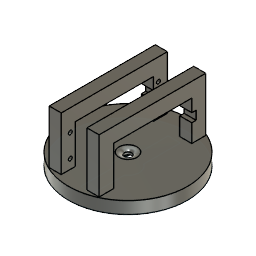
Circle (Autodesk Fusion 360 design; units mm, degrees)
Autodesk Fusion 360 part; units mm, degrees
sketch "Sketch1" plane through (0, 0, 0) normal (0, 0, 1) x (1, 0, 0)
  circle A0 centre (0, 0) radius 31.115
  dimension "d1" = 62.23
  constraint coincident A0.centre origin
  measures "d1" diameter of A0
extrude "Extrude1" add sketch "Sketch1" along normal blind 7.62 contours A0 picked at (8.859186, 0.873231) makes body 1
sketch "Sketch2" plane through (0, 0, 7.62) normal (0, 0, 1) x (-1, 0, 0)
  circle A0 centre (0, 0) radius 31.115
  circle A1 centre (0, 0) radius 1.905
  dimension "d4" = 3.81
  constraint coincident A0.centre A1.centre
  measures "d4" diameter of A1
extrude "Extrude2" cut sketch "Sketch2" against normal blind 27.94 contours A1 picked at (-0.336742, 0.293155) bodies 1
extrude "Extrude3" cut 1 faces at (21.255398, -1.640459, 7.62) along direction (0, 0, -1) blind 1.27 on bodies 1 bodies 1
sketch "Sketch3" plane through (0, 0, 6.35) normal (0, 0, 1) x (-1, 0, 0)
  circle A0 centre (0, 0) radius 1.905
  circle A1 centre (0, 0) radius 31.115
  line L0 (3.173876, -26.67) -> (-3.176124, -26.67)
  line L1 (3.173876, -26.67) -> (3.173876, 24.13)
  line L2 (-3.176124, -26.67) -> (-3.176124, 21.675024)
  line L3 (3.173876, 24.13) -> (-3.176124, 24.13)
  line L4 (-3.176124, 24.13) -> (-3.176124, 21.675024)
  dimension "d9" = 50.8
  constraint horizontal L0
  constraint perpendicular L0 L1
  constraint perpendicular L0 L2
  constraint perpendicular L2 L3
  constraint perpendicular L3 L4
extrude "Extrude4" cut sketch "Sketch3" against normal blind 5.08 contours L0 L1 L2 L3 L4 picked at (-0.048203, -18.413224) bodies 1
sketch "Sketch4" plane through (0, 0, 6.35) normal (0, 0, 1) x (-1, 0, 0)
  line L0 (-3.176124, 24.13) -> (3.173876, 24.13)
  line L1 (3.173876, 24.13) -> (3.173876, -26.67)
  line L2 (3.173876, -26.67) -> (-3.176124, -26.67)
  line L3 (-3.176124, -26.67) -> (-3.176124, 24.13)
  circle A0 centre (0, 0) radius 31.115
  circle A1 centre (0, 0) radius 5.08
  constraint coincident A0.centre A1.centre
extrude "Extrude5" cut sketch "Sketch4" against normal blind 5.08 contours L3 A1 | L1 A1 picked at (-4.180187, 0) picked at (3.3588, -1.150052) bodies 1
extrude "Extrude6" cut 1 faces at (-3.173876, -10.687649, 4.656667) along direction (-1, 0, 0) blind 2.54 on bodies 1 bodies 1
extrude "Extrude7" cut 1 faces at (-3.173876, 11.534316, 2.963333) along direction (-1, 0, 0) blind 2.54 on bodies 1 bodies 1
extrude "Extrude8" cut 1 faces at (3.176124, 19.101558, 4.656667) along direction (1, 0, 0) blind 2.54 on bodies 1 bodies 1
extrude "Extrude9" cut 1 faces at (3.176124, -17.408225, 4.656667) along direction (1, 0, 0) blind 2.54 on bodies 1 bodies 1
sketch "Sketch5" plane through (0, 0, 6.35) normal (0, 0, 1) x (-1, 0, 0)
  circle A0 centre (0, 0) radius 31.115
  line L0 (-3.176124, 3.964673) -> (-5.716124, 3.964673)
  line L1 (-5.716124, 3.964673) -> (-5.716124, 24.13)
  line L2 (-5.716124, 24.13) -> (5.713876, 24.13)
  line L3 (5.713876, 24.13) -> (5.713876, 3.966474)
  line L4 (5.713876, 3.966474) -> (3.173876, 3.966474)
  arc A1 (3.173876, -3.966474) -> (3.173876, 3.966474) centre (0, 0) ccw
  line L5 (3.173876, -3.966474) -> (5.713876, -3.966474)
  line L6 (5.713876, -3.966474) -> (5.713876, -26.67)
  line L7 (5.713876, -26.67) -> (-5.716124, -26.67)
  line L8 (-5.716124, -26.67) -> (-5.716124, -3.964673)
  line L9 (-5.716124, -3.964673) -> (-3.176124, -3.964673)
  arc A2 (-3.176124, 3.964673) -> (-3.176124, -3.964673) centre (0, 0) ccw
  circle A3 centre (0, 0) radius 7.62
  constraint coincident A0.centre A1.centre
extrude "Extrude10" cut sketch "Sketch5" against normal blind 5.08 contours L0 L1 L8 L9 A2 A3 | L3 L4 A1 L5 L6 A3 picked at (-5.736875, 3.121518) picked at (5.735631, -3.123168) bodies 1
extrude "Extrude11" add 1 faces at (1.906124, 26.67, 2.963333) along direction (0, -1, 0) blind 2.54 on bodies 1 bodies 1
extrude "Extrude12" add 1 faces at (-1.903876, -24.13, 2.963333) along direction (0, 1, 0) blind 2.54 on bodies 1 bodies 1
move_body "Move1" bodies 1 to x (-1, 0, 0) y (0, 1, 0) z (0, 0, -1) at (24.534657, 0, 12.7)
extrude "Extrude13" add 1 faces at (30.248533, -10.557621, 8.043333) along direction (-1, 0, 0) blind 0.127 on bodies 1 bodies 1
extrude "Extrude14" add 1 faces at (30.248533, 17.767144, 8.043333) along direction (-1, 0, 0) blind 0.127 on bodies 1 bodies 1
extrude "Extrude15" add 1 faces at (18.818533, 11.402588, 9.736666) along direction (1, 0, 0) blind 0.127 on bodies 1 bodies 1
extrude "Extrude16" add 1 faces at (18.818533, -16.072961, 9.736666) along direction (1, 0, 0) blind 0.127 on bodies 1 bodies 1
sketch "Sketch6" plane through (0, 0, 0) normal (1, 0, 0) x (0, 1, 0)
sketch "Sketch7" plane through (0, 0, 0) normal (1, 0, 0) x (0, 1, 0)
move_body "Move2" bodies 1 to x (1, 0, 0) y (0, 1, 0) z (0, 0, 1) at (-20.32, 0, -7.62)
sketch "Sketch9" plane through (0, 0, 0) normal (0, 1, 0) x (1, 0, 0)
sketch "Sketch10" plane through (0, 0, 0) normal (0, 1, 0) x (1, 0, 0)
sketch "Sketch11" plane through (0, 0, 0) normal (0, 1, 0) x (1, 0, 0)
sketch "Sketch12" plane through (0, 0, 0) normal (0, 1, 0) x (1, 0, 0)
  line L0 (0, -38.100001) -> (40.894, -38.100001)
  line L1 (40.894, -38.100001) -> (40.894, -17.526001)
  line L2 (40.894, -17.526001) -> (0, -17.526001)
  line L3 (0, -17.526001) -> (0, -38.100001)
  circle A0 centre (20.447, -27.813001) radius 27.94
  dimension "d39" = 40.894
  dimension "d40" = 20.574
  dimension "d41" = 55.88
  constraint horizontal L0
  constraint vertical L1
  constraint horizontal L2
  constraint vertical L3
  measures "d41" diameter of A0
move_body "Move3" bodies 1 to x (1, 0, 0) y (0, 1, 0) z (0, 0, 1) at (-55.88, 0, 0)
sketch "Sketch13" plane through (0, 0, 0) normal (1, 0, 0) x (0, 1, 0)
sketch "Sketch14" plane through (0, 0, 0) normal (1, 0, 0) x (0, 1, 0)
sketch "Sketch15" plane through (0, 0, 0) normal (1, 0, 0) x (0, 1, 0)
  line L0 (127.000004, 38.100001) -> (167.894004, 38.100001)
  line L1 (167.894004, 38.100001) -> (167.894004, 17.526001)
  line L2 (167.894004, 17.526001) -> (127.000004, 17.526001)
  line L3 (127.000004, 17.526001) -> (127.000004, 38.100001)
  circle A0 centre (147.447004, 27.813001) radius 27.94
  dimension "d44" = 40.894
  dimension "d45" = 20.574
  dimension "d46" = 55.88
  constraint horizontal L0
  constraint vertical L1
  constraint horizontal L2
  constraint vertical L3
  measures "d46" diameter of A0
sketch "Sketch16" plane through (0, 0, 0) normal (1, 0, 0) x (0, 1, 0)
sketch "Sketch17" plane through (0, 0, 0) normal (1, 0, 0) x (0, 1, 0)
  line L0 (76.200002, 50.800002) -> (117.094002, 50.800002)
  line L1 (117.094002, 50.800002) -> (117.094002, 30.226002)
  line L2 (117.094002, 30.226002) -> (76.200002, 30.226002)
  line L3 (76.200002, 30.226002) -> (76.200002, 50.800002)
  line L4 (96.647002, 40.513002) -> (68.580002, 40.513002)
  line L5 (68.580002, 40.513002) -> (68.580002, 58.420002)
  line L6 (68.580002, 58.420002) -> (96.647002, 58.420002)
  line L7 (96.647002, 58.420002) -> (96.647002, 40.513002)
  line L8 (96.647002, 40.513002) -> (124.460004, 40.513002)
  line L9 (124.460004, 40.513002) -> (124.460004, 22.860001)
  line L10 (124.460004, 22.860001) -> (96.647002, 22.860001)
  line L11 (96.647002, 22.860001) -> (96.647002, 40.513002)
  line L12 (68.580002, 58.420002) -> (124.460004, 58.420002)
  line L13 (124.460004, 58.420002) -> (124.460004, 22.860001)
  line L14 (124.460004, 22.860001) -> (68.580002, 22.860001)
  line L15 (68.580002, 22.860001) -> (68.580002, 58.420002)
  dimension "d53" = 40.894
  dimension "d54" = 20.574
  constraint horizontal L0
  constraint vertical L1
  constraint horizontal L2
  constraint vertical L3
  constraint horizontal L4
  constraint vertical L5
  constraint horizontal L6
  constraint vertical L7
  constraint horizontal L8
  constraint vertical L9
  constraint horizontal L10
  constraint vertical L11
  constraint horizontal L12
  constraint vertical L13
  constraint horizontal L14
  constraint vertical L15
extrude "Extrude21" add sketch "Sketch17" against normal blind 7.62 separate body contours L0 L3 L4 L5 L6 L7 L12 L15 | L0 L1 L7 L8 L12 L13 | L2 L3 L4 L11 L14 L15 | L1 L2 L8 L9 L10 L11 L13 L14 picked at (80.475669, 55.880002) picked at (112.73367, 55.880002) picked at (80.475669, 25.315334) picked at (112.73367, 25.315334) makes body 2
extrude "Extrude22" cut 1 faces at (0, 80.475669, 55.880002) along direction (-1, 0, 0) blind 2.54 on bodies 2 bodies 2
move_body "Move22" bodies 2 to x (1, 0, 0) y (0, 1, 0) z (0, 0, 1) at (-38.1, -96.52, -22.86)
move_body "Move23" bodies 2 to x (1, 0, 0) y (0, 1, 0) z (0, 0, 1) at (0, 0, -2.54)
move_body "Move24" bodies 2 to x (1, 0, 0) y (0, 1, 0) z (0, 0, 1) at (0, 0, 1.27)
sketch "Sketch18" plane through (0, 0, 0) normal (0, 0, 1) x (1, 0, 0)
move_body "Move25" bodies 2 to x (1, 0, 0) y (0, 1, 0) z (0, 0, 1) at (2.54, 0, 0)
move_body "Move26" bodies 2 to x (1, 0, 0) y (0, 1, 0) z (0, 0, 1) at (0, 0, 1.27)
move_body "Move27" bodies 2 to x (1, 0, 0) y (0, 1, 0) z (0, 0, 1) at (-1.27, 0, 0)
move_body "Move28" bodies 2 to x (1, 0, 0) y (0, 1, 0) z (0, 0, 1) at (0.508, 0, 0)
move_body "Move29" bodies 2 to x (1, 0, 0) y (0, 1, 0) z (0, 0, 1) at (0, 0, -1.27)
move_body "Move30" bodies 2 to x (1, 0, 0) y (0, 1, 0) z (0, 0, 1) at (0, 0, -1.016)
extrude "Extrude23" cut 1 faces at (-40.555333, 9.313337, -2.285999) along direction (0, 0, 1) blind 2.54 on bodies 2 bodies 1 2
extrude "Extrude24" add 1 faces at (-43.942, 9.313337, -0.762) along direction (1, 0, 0) blind 5.08 on bodies 1 bodies 1 2
sketch "Sketch19" plane through (0, 0, 0) normal (1, 0, 0) x (0, 1, 0)
  line L0 (50.800002, 25.400001) -> (91.694002, 25.400001)
  line L1 (91.694002, 25.400001) -> (91.694002, 4.826001)
  line L2 (91.694002, 4.826001) -> (50.800002, 4.826001)
  line L3 (50.800002, 4.826001) -> (50.800002, 25.400001)
  line L4 (50.800002, 21.590001) -> (43.434002, 21.590001)
  line L5 (57.150002, 25.400001) -> (57.150002, 33.020001)
  line L6 (57.150002, 33.020001) -> (43.434002, 33.020001)
  line L7 (43.180001, 23.50981) -> (43.180001, 22.860001)
  line L8 (43.434002, 21.590001) -> (43.434002, 33.020001)
  line L9 (91.694002, 4.826001) -> (99.06, 4.826001)
  line L10 (91.694002, 25.400001) -> (91.694002, 33.020001)
  line L11 (91.694002, 20.027669) -> (99.060002, 20.027669)
  line L12 (91.694002, 33.020001) -> (99.060003, 33.020001)
  line L13 (99.060003, 33.020001) -> (99.060002, 20.027669)
  line L14 (43.434002, 33.020001) -> (99.06, 33.020001)
  line L15 (99.06, 33.020001) -> (99.06, 4.826001)
  line L16 (99.06, 4.826001) -> (43.434002, 4.826001)
  line L17 (43.434002, 4.826001) -> (43.434002, 33.020001)
  dimension "d63" = 40.894
  dimension "d64" = 20.574
  dimension "d65" = 7.366
  dimension "d66" = 7.62
  dimension "d67" = 7.62
  dimension "d68" = 7.366
  constraint horizontal L0
  constraint vertical L1
  constraint horizontal L2
  constraint vertical L3
  constraint perpendicular L3 L4
  constraint perpendicular L0 L5
  constraint perpendicular L5 L6
  constraint perpendicular L4 L7
  constraint perpendicular L6 L8
  constraint perpendicular L1 L9
  constraint perpendicular L0 L10
  constraint perpendicular L1 L11
  constraint perpendicular L10 L12
  constraint horizontal L14
  constraint vertical L15
  constraint horizontal L16
  constraint vertical L17
extrude "Extrude25" add sketch "Sketch19" against normal blind 2.54 separate body contours L0 L3 L4 L5 L6 L8 L14 L17 | L0 L5 L10 L14 | L3 L4 L16 L17 | L1 L10 L11 L12 L13 L14 L15 | L1 L9 L11 L15 L16 picked at (50.461335, 30.480001) picked at (68.664668, 30.480001) picked at (45.889335, 10.414001) picked at (96.604669, 26.149223) picked at (96.604668, 14.960446) makes body 3
extrude "Extrude26" add 1 faces at (0, 80.179335, 27.940001) along direction (1, 0, 0) blind 2.54 on bodies 3 bodies 3
move_body "Move31" bodies 3 to x (1, 0, 0) y (0, 1, 0) z (0, 0, 1) at (-63.5, -71.12, 0)
move_body "Move32" bodies 3 to x (1, 0, 0) y (0, 1, 0) z (0, 0, 1) at (2.54, 0, 0)
move_body "Move33" bodies 3 to x (1, 0, 0) y (0, 1, 0) z (0, 0, 1) at (-1.27, 0, 0)
move_body "Move34" bodies 3 to x (1, 0, 0) y (0, 1, 0) z (0, 0, 1) at (-0.508, 0, 0)
sketch "Sketch20" plane through (0, 0, 0) normal (1, 0, 0) x (0, 1, 0)
  circle A0 through (24.20431, 9.927898, -65.278) (22.68031, 10.807779, -65.278) (22.68031, 9.048016, -65.278)
  circle A1 through (-21.917009, 21.767801, -65.267431) (-23.441009, 22.647682, -65.267431) (-23.441009, 20.887919, -65.267431)
  circle A2 through (-21.9202, 9.931401, -65.2526) (-23.4442, 10.811282, -65.2526) (-23.4442, 9.051519, -65.2526)
  circle A3 through (24.2062, 21.767801, -65.278) (22.6822, 22.647682, -65.278) (22.6822, 20.887919, -65.278)
  dimension "d73" = 2.032
  dimension "d74" = 2.032
  dimension "d75" = 2.032
  dimension "d76" = 2.032
extrude "Extrude27" cut sketch "Sketch20" along normal blind 7.62 contours A0 | A3 in plane through (-65.278, 0, 0) normal (1, 0, 0) picked at (-65.278, 23.163002, 10.176766) picked at (-65.278, 22.94194, 21.537449) bodies 3
sketch "Sketch21" plane through (-65.278, 0, 0) normal (-1, 0, 0) x (0, -1, 0)
  circle A0 centre (-23.1902, 21.767801) radius 1.016
  circle A1 centre (-23.18831, 9.927898) radius 1.016
  line L0 (20.319998, 25.400001) -> (20.319998, 4.826001)
  line L1 (20.319998, 4.826001) -> (27.685998, 4.826001)
  line L2 (27.685998, 4.826001) -> (27.685998, 33.020001)
  line L3 (27.685998, 33.020001) -> (-27.94, 33.020001)
  line L4 (-27.94, 33.020001) -> (-27.94, 4.826001)
  line L5 (-27.94, 4.826001) -> (-20.574002, 4.826001)
  line L6 (-20.574002, 4.826001) -> (-20.574002, 25.400001)
  line L7 (-20.574002, 25.400001) -> (20.319998, 25.400001)
  circle A2 centre (22.936201, 21.767801) radius 1.016
  dimension "d79" = 2.032
  measures "d79" diameter of A2
sketch "Sketch22" plane through (-65.278, 0, 0) normal (-1, 0, 0) x (0, -1, 0)
extrude "Extrude28" cut sketch "Sketch21" against normal blind 10.16 contours A2 picked at (22.909209, 22.083057) bodies 3
sketch "Sketch23" plane through (-65.278, 0, 0) normal (-1, 0, 0) x (0, -1, 0)
  circle A0 centre (22.936201, 21.767801) radius 1.016
  circle A1 centre (-23.1902, 21.767801) radius 1.016
  circle A2 centre (-23.18831, 9.927898) radius 1.016
  line L0 (20.319998, 25.400001) -> (20.319998, 4.826001)
  line L1 (20.319998, 4.826001) -> (27.685998, 4.826001)
  line L2 (27.685998, 4.826001) -> (27.685998, 33.020001)
  line L3 (27.685998, 33.020001) -> (-27.94, 33.020001)
  line L4 (-27.94, 33.020001) -> (-27.94, 4.826001)
  line L5 (-27.94, 4.826001) -> (-20.574002, 4.826001)
  line L6 (-20.574002, 4.826001) -> (-20.574002, 25.400001)
  line L7 (-20.574002, 25.400001) -> (20.319998, 25.400001)
  circle A3 centre (22.934741, 9.940172) radius 1.016
  dimension "d82" = 2.032
  measures "d82" diameter of A3
extrude "Extrude29" cut sketch "Sketch23" against normal blind 8.89 contours A3 picked at (23.476333, 9.720291) bodies 3
sketch "Sketch24" plane through (-65.278, 0, 0) normal (-1, 0, 0) x (0, -1, 0)
  circle A0 centre (22.934741, 9.940172) radius 1.016
  circle A1 centre (22.936201, 21.767801) radius 1.016
  circle A2 centre (-23.1902, 21.767801) radius 1.016
  circle A3 centre (-23.18831, 9.927898) radius 1.016
  line L0 (20.319998, 25.400001) -> (20.319998, 4.826001)
  line L1 (20.319998, 4.826001) -> (27.685998, 4.826001)
  line L2 (27.685998, 4.826001) -> (27.685998, 33.020001)
  line L3 (27.685998, 33.020001) -> (-27.94, 33.020001)
  line L4 (-27.94, 33.020001) -> (-27.94, 4.826001)
  line L5 (-27.94, 4.826001) -> (-20.574002, 4.826001)
  line L6 (-20.574002, 4.826001) -> (-20.574002, 25.400001)
  line L7 (-20.574002, 25.400001) -> (20.319998, 25.400001)
  line L8 (-20.574, 19.05) -> (-22.86, 19.05)
  line L9 (-22.86, 19.05) -> (-22.86, 14.478)
  line L10 (-22.86, 14.478) -> (-20.574002, 14.478)
  constraint coincident L6 L8.start
  constraint perpendicular L6 L8
  constraint perpendicular L8 L9
  constraint perpendicular L6 L10
extrude "Extrude30" cut sketch "Sketch24" against normal blind 5.08 contours L6 L8 L9 L10 picked at (-22.098, 17.526) bodies 3
sketch "Sketch25" plane through (-43.942, 0, 0) normal (-1, 0, 0) x (0, -1, 0)
  line L0 (20.319998, 5.080002) -> (27.939998, 5.08)
  line L1 (27.939998, 5.08) -> (27.939998, 33.274002)
  line L2 (27.939998, 33.274002) -> (-27.940004, 33.274002)
  line L3 (-27.940004, 33.274002) -> (-27.940004, 5.08)
  line L4 (-27.940004, 5.08) -> (-20.574002, 5.080002)
  line L5 (-20.574002, 5.080002) -> (-20.574002, 25.654002)
  line L6 (-20.574002, 25.654002) -> (20.319998, 25.654002)
  line L7 (20.319998, 25.654002) -> (20.319998, 5.080002)
  line L8 (-20.574, 19.05) -> (-22.86, 19.05)
  line L9 (-22.86, 19.05) -> (-22.86, 14.478)
  line L10 (-22.86, 14.478) -> (-20.574002, 14.478)
  constraint coincident L5 L8.start
  constraint perpendicular L5 L8
  constraint perpendicular L8 L9
  constraint perpendicular L5 L10
extrude "Extrude31" cut sketch "Sketch25" against normal blind 27.94 contours L5 L8 L9 L10 picked at (-22.098001, 17.526) bodies 1
extrude "Extrude32" add 1 faces at (-60.198, 6.942669, 30.480001) along direction (1, 0, 0) blind 1.27 on bodies 3 bodies 1 3
extrude "Extrude33" add 1 faces at (-43.942, -6.77333, 30.734002) along direction (-1, 0, 0) blind 1.27 on bodies 1 bodies 1
fillet "Fillet1" radius 3.81 1 edges at (-53.441427, 0.688877, 5.08) on bodies 1
extrude "Extrude34" add 1 faces at (-57.254467, 11.402588, 0.423333) along direction (1, 0, 0) blind 2.54 on bodies 1 bodies 1
extrude "Extrude35" add 1 faces at (-46.078467, 17.767144, 0.423333) along direction (-1, 0, 0) blind 2.54 on bodies 1 bodies 1
extrude "Extrude36" add 1 faces at (-46.078467, -10.557621, 0.423333) along direction (-1, 0, 0) blind 2.54 on bodies 1 bodies 1
extrude "Extrude37" add 1 faces at (-57.254467, -16.072961, 2.116666) along direction (1, 0, 0) blind 2.54 on bodies 1 bodies 1
sketch "Sketch26" plane through (0, 0, 3.81) normal (0, 0, -1) x (1, 0, 0)
  circle A0 centre (-51.665343, 0) radius 1.905
  line L0 (-54.714467, 21.59) -> (-54.714467, 5.038881)
  line L1 (-54.714467, 5.038881) -> (-57.381467, 5.038881)
  arc A1 (-57.381467, 5.038881) -> (-57.381467, -5.038881) centre (-51.665343, 0) ccw
  line L2 (-57.381467, -5.038881) -> (-54.714467, -5.038881)
  line L3 (-54.714467, -5.038881) -> (-54.714467, -24.13)
  line L4 (-54.714467, -24.13) -> (-48.618467, -24.13)
  line L5 (-48.618467, -24.13) -> (-48.618467, -5.041431)
  line L6 (-48.618467, -5.041431) -> (-45.951467, -5.041431)
  arc A2 (-45.951467, -5.041431) -> (-45.951467, 5.041431) centre (-51.665343, 0) ccw
  line L7 (-45.951467, 5.041431) -> (-48.618467, 5.041431)
  line L8 (-48.618467, 5.041431) -> (-48.618467, 21.59)
  line L9 (-48.618467, 21.59) -> (-54.714467, 21.59)
  circle A3 centre (-51.665343, 0) radius 7.215342
  constraint concentric A0 A3
extrude "Extrude38" add sketch "Sketch26" along normal blind 2.54 contours L0 L1 L2 L3 L5 L6 L7 L8 A3 picked at (-48.032767, 3.224312) bodies 1
extrude "Extrude39" add 1 faces at (-53.077996, 4.692535, 1.27) along direction (0, 0, -1) blind 2.54 on bodies 1 bodies 1
extrude "Extrude40" add 1 faces at (-44.327006, 0, 3.81) along direction (0, 0, -1) blind 5.08 on bodies 1 bodies 1
extrude "Extrude41" add 1 faces at (-59.003696, 0, 3.81) along direction (0, 0, -1) blind 5.08 on bodies 1 bodies 1
sketch "Sketch27" plane through (0, 0, -1.27) normal (0, 0, -1) x (1, 0, 0)
  line L0 (-54.714467, 6.539419) -> (-54.714467, 21.59)
  line L1 (-54.714467, 21.59) -> (-48.618467, 21.59)
  line L2 (-48.618467, 21.59) -> (-48.618467, 6.540467)
  arc A0 (-48.618467, 6.540467) -> (-54.714467, 6.539419) centre (-51.665343, 0) ccw
  circle A1 centre (-51.665343, 0) radius 1.905
  arc A2 (-54.714467, -6.539419) -> (-48.618467, -6.540467) centre (-51.665343, 0) ccw
  line L3 (-48.618467, -6.540467) -> (-48.618467, -24.13)
  line L4 (-48.618467, -24.13) -> (-54.714467, -24.13)
  line L5 (-54.714467, -24.13) -> (-54.714467, -6.539419)
  circle A3 centre (-51.665343, 0) radius 31.115
  circle A4 centre (-51.665343, 0) radius 5.945342
  constraint concentric A0 A4
extrude "Extrude42" cut sketch "Sketch27" against normal blind 3.81 contours A4 picked at (-47.088917, -0.295369) bodies 1
sketch "Sketch28" plane through (0, 0, -1.27) normal (0, 0, -1) x (1, 0, 0)
  circle A0 centre (-51.665343, 0) radius 5.945342
  line L0 (-54.714467, 6.539419) -> (-54.714467, 21.59)
  line L1 (-54.714467, 21.59) -> (-48.618467, 21.59)
  line L2 (-48.618467, 21.59) -> (-48.618467, 6.540467)
  arc A1 (-48.618467, 6.540467) -> (-54.714467, 6.539419) centre (-51.665343, 0) ccw
  arc A2 (-54.714467, -6.539419) -> (-48.618467, -6.540467) centre (-51.665343, 0) ccw
  line L3 (-48.618467, -6.540467) -> (-48.618467, -24.13)
  line L4 (-48.618467, -24.13) -> (-54.714467, -24.13)
  line L5 (-54.714467, -24.13) -> (-54.714467, -6.539419)
  circle A3 centre (-51.665343, 0) radius 31.115
  line L6 (-54.714467, 6.539419) -> (-54.714467, 5.103913)
  line L7 (-54.714467, 5.103913) -> (-48.616219, 5.103913)
  line L8 (-48.618467, 6.540467) -> (-48.616219, 5.103913)
  line L9 (-54.714467, -6.539419) -> (-54.714467, -5.103913)
  line L10 (-54.714467, -5.103913) -> (-48.616219, -5.103913)
  line L11 (-48.618467, -6.540467) -> (-48.616219, -5.103913)
  line L12 (-54.714467, -6.539419) -> (-48.618467, -6.540467)
  line L13 (-54.714467, 6.539419) -> (-48.618467, 6.540467)
  constraint parallel L0 L6
  constraint perpendicular L6 L7
  constraint perpendicular L7 L9
  constraint perpendicular L9 L10
extrude "Extrude43" cut sketch "Sketch28" against normal blind 3.81 contours A0 L6 L8 L13 | A0 L9 L11 L12 | A1 L13 | A2 L12 picked at (-51.666093, 6.341742) picked at (-51.666093, -6.341742) picked at (-52.014917, 6.739645) picked at (-52.35597, -6.664011) bodies 1
extrude "Extrude44" add 1 faces at (-51.666506, 18.49178, 3.81) along direction (0, 0, -1) blind 1.27 on bodies 1 bodies 1
extrude "Extrude45" add 1 faces at (-51.666506, -16.798447, 3.81) along direction (0, 0, -1) blind 1.27 on bodies 1 bodies 1
extrude "Extrude46" cut 1 faces at (-54.714467, 11.445942, 1.27) along direction (-1, 0, 0) blind 0.127 on bodies 1 bodies 1
extrude "Extrude47" cut 1 faces at (-48.618467, 12.403644, 1.27) along direction (1, 0, 0) blind 0.127 on bodies 1 bodies 1
extrude "Extrude48" cut 1 faces at (-54.756801, 5.103913, 0) along direction (0, -1, 0) blind 0.762 on bodies 1 bodies 1
extrude "Extrude49" cut 1 faces at (-48.576134, 6.540467, 1.27) along direction (0, -1, 0) blind 1.524 on bodies 1 bodies 1
extrude "Extrude50" cut 1 faces at (-54.714467, -10.599275, 1.27) along direction (-1, 0, 0) blind 0.127 on bodies 1 bodies 1
extrude "Extrude51" cut 1 faces at (-48.618467, -16.573489, 1.27) along direction (1, 0, 0) blind 0.127 on bodies 1 bodies 1
extrude "Extrude52" cut 1 faces at (-48.576134, -6.540467, 0) along direction (0, 1, 0) blind 2.032 on bodies 1 bodies 1
extrude "Extrude53" cut 1 faces at (-54.756801, -5.103913, 0) along direction (0, 1, 0) blind 1.016 on bodies 1 bodies 1
sketch "Sketch29" plane through (0, 0, -1.27) normal (0, 0, -1) x (1, 0, 0)
  line L0 (-54.841467, 5.025865) -> (-54.841467, 21.59)
  line L1 (-54.841467, 21.59) -> (-48.491467, 21.59)
  line L2 (-48.491467, 21.59) -> (-48.491467, 5.027286)
  arc A0 (-48.491467, -5.027286) -> (-48.491467, 5.027286) centre (-51.665343, 0) ccw
  line L3 (-48.491467, -5.027286) -> (-48.491467, -24.13)
  line L4 (-48.491467, -24.13) -> (-54.841467, -24.13)
  line L5 (-54.841467, -24.13) -> (-54.841467, -5.025865)
  arc A1 (-54.841467, 5.025865) -> (-54.841467, -5.025865) centre (-51.665343, 0) ccw
  circle A2 centre (-51.665343, 0) radius 31.115
sketch "Sketch30" plane through (0, 0, -1.27) normal (0, 0, -1) x (1, 0, 0)
sketch "Sketch31" plane through (0, 0, -1.27) normal (0, 0, -1) x (1, 0, 0)
sketch "Sketch32" plane through (0, 0, -1.27) normal (0, 0, -1) x (1, 0, 0)
sketch "Sketch33" plane through (0, 0, -1.27) normal (0, 0, -1) x (1, 0, 0)
  circle A0 centre (-51.688999, 0) radius 6.2865
  dimension "d135" = 12.573
  measures "d135" diameter of A0
extrude "Extrude54" cut sketch "Sketch33" against normal blind 3.81 contours A0 picked at (-49.686597, 1.200747) bodies 1
sketch "Sketch34" plane through (0, 0, -1.27) normal (0, 0, -1) x (1, 0, 0)
  line L0 (-54.863999, 21.59) -> (-48.513999, 21.59)
  line L1 (-48.513999, 21.59) -> (-48.513999, 21.082)
  line L2 (-48.513999, 21.082) -> (-54.863999, 21.082)
  line L3 (-54.863999, 21.082) -> (-54.863999, 21.59)
  line L4 (-51.688999, 24.099104) -> (-56.235599, 24.099104)
  line L5 (-56.235599, 24.099104) -> (-47.142399, 24.099104)
  line L6 (-56.235599, 24.099104) -> (-56.235599, 4.064)
  line L7 (-56.235599, 4.064) -> (-47.142399, 4.064)
  line L8 (-47.142399, 4.064) -> (-47.142399, 24.099104)
  line L9 (-56.235599, 4.064) -> (-56.235599, -24.130001)
  line L10 (-56.235599, -24.130001) -> (-47.142399, -24.130001)
  line L11 (-47.142399, -24.130001) -> (-47.142399, 4.064)
  dimension "d138" = 4.5466
  dimension "d139" = 9.0932
  constraint horizontal L0
  constraint vertical L1
  constraint horizontal L2
  constraint vertical L3
  constraint parallel L0 L4
  constraint parallel L4 L5
  constraint perpendicular L5 L6
  constraint perpendicular L6 L7
  constraint perpendicular L5 L8
  constraint perpendicular L7 L9
  constraint perpendicular L8 L10
  constraint perpendicular L7 L11
extrude "Extrude55" cut sketch "Sketch34" against normal blind 3.81 contours L7 L9 L10 L11 picked at (-53.204533, -14.732001) bodies 1
sketch "Sketch35" plane through (0, 0, -1.27) normal (0, 0, -1) x (1, 0, 0)
  line L0 (-56.2356, -3.355685) -> (-56.2356, 21.59)
  line L1 (-56.2356, 21.59) -> (-47.1424, 21.59)
  line L2 (-47.1424, 21.59) -> (-47.1424, -3.355685)
  line L3 (-47.1424, -3.355685) -> (-56.2356, -3.355685)
  dimension "d142" = 9.0932
  constraint vertical L0
  constraint perpendicular L0 L1
  constraint perpendicular L1 L2
  constraint perpendicular L2 L3
  measures "d142" distance of L0.end L1.end
extrude "Extrude56" cut sketch "Sketch35" against normal blind 3.81 contours L0 L1 L2 L3 picked at (-50.173467, 13.274771) bodies 1
